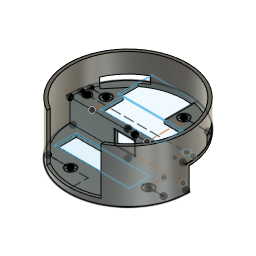
Echo_dev_dock_v1 (Autodesk Fusion 360 design; units mm, degrees)
Autodesk Fusion 360 part; units mm, degrees
sketch "Sketch1" plane through (0, 0, 0) normal (0, 0, 1) x (1, 0, 0)
  circle A0 centre (0, 0) radius 37.65
  line L0 (37.65, 1) -> (-37.65, 1)
  line L1 (-37.65, 1) -> (-37.65, -1)
  line L2 (-37.65, -1) -> (37.65, -1)
  line L3 (37.65, -1) -> (37.65, 1)
  line L4 (37.65, 1) -> (-37.65, -1) construction
  line L5 (-37.65, 1) -> (37.65, -1) construction
  dimension "d1" = 75.3
  dimension "d13" = 75.3
  dimension "d14" = 2
  constraint coincident A0.centre origin
  constraint horizontal L0
  constraint perpendicular L0 L1
  constraint parallel L0 L2
  constraint parallel L1 L3
  constraint coincident L4 A0.centre
  constraint coincident L5 A0.centre
  measures "d1" diameter of A0
  measures "d13" distance of L1.end L2.end
  measures "d14" distance of L0.end L1.end
extrude "Extrude1" add sketch "Sketch1" along normal blind 17 contours A0 L0 L2 | A0 L0 | A0 L2 makes body 1
sketch "Sketch2" plane through (0, 0, 17) normal (0, 0, 1) x (-1, 0, 0)
  circle A0 centre (0, 0) radius 37.65
  line L0 (-37.65, 1) -> (37.65, 1)
  line L1 (37.65, 1) -> (37.65, -1)
  line L2 (37.65, -1) -> (-37.65, -1)
  line L3 (-37.65, -1) -> (-37.65, 1)
  line L4 (-37.65, 1) -> (37.65, -1) construction
  line L5 (37.65, 1) -> (-37.65, -1) construction
  dimension "d4" = 75.3
  dimension "d5" = 2
  constraint horizontal L0
  constraint perpendicular L0 L1
  constraint parallel L0 L2
  constraint parallel L1 L3
  constraint coincident L4 A0.centre
  constraint coincident L5 A0.centre
  constraint coincident A0.centre origin
  measures "d4" distance of L1.end L2.end
  measures "d5" distance of L0.end L1.end
ref_plane "WorkPlane3" through (0, 19.325, 0) normal (0, 0, 1) x (-1, 0, 0)
extrude "Extrude2" cut sketch "Sketch2" against normal blind 15 contours A0 L0 bodies 1
ref_plane "WorkPlane1" through (0, 19.325, 0) normal (0, 0, 1) x (-1, 0, 0)
sketch "Sketch3" plane through (0, 19.325, 0) normal (0, 0, 1) x (1, 0, 0)
ref_plane "WorkPlane2" through (0, 19.325, 0) normal (0, 0, 1) x (-1, 0, 0)
sketch "Sketch4" plane through (0, 19.325, 0) normal (0, 0, 1) x (1, 0, 0)
sketch "Sketch5" plane through (0, 19.325, 0) normal (0, 0, 1) x (1, 0, 0)
ref_plane "WorkPlane4" through (0, 19.325, 0) normal (0, 0, 1) x (-1, 0, 0)
sketch "Sketch6" plane through (0, 19.325, 0) normal (0, 0, 1) x (1, 0, 0)
  line L0 (37.65, -18.3) -> (-37.65, -18.3)
  line L1 (-37.65, -18.3) -> (-37.65, -20.3)
  line L2 (-37.65, -20.3) -> (37.65, -20.3)
  line L3 (37.65, -20.3) -> (37.65, -18.3)
  line L4 (37.65, -18.3) -> (-37.65, -20.3) construction
  line L5 (-37.65, -18.3) -> (37.65, -20.3) construction
  point P0 (0, -19.3)
  dimension "d12" = 75.3
  constraint horizontal L0
  constraint perpendicular L0 L1
  constraint parallel L0 L2
  constraint parallel L1 L3
  constraint coincident L4 P0
  constraint coincident L5 P0
  measures "d12" distance of L1.end L2.end
extrude "Extrude3" cut sketch "Sketch1" along normal blind 15 contours A0 L0 bodies 1
sketch "Sketch8" plane through (0, 0, 2) normal (0, 0, 1) x (-1, 0, 0)
  arc A0 (37.6367, 1) -> (-37.6367, 1) centre (0, 0) ccw
  line L0 (-37.6367, 1) -> (37.6367, 1)
  line L1 (0, 37.65) -> (0, 26.65) construction
  line L2 (0, 26.65) -> (26.5951, 26.65) construction
  line L3 (26.5951, 26.65) -> (11.5951, 26.65) construction
  circle A1 centre (11.5951, 26.65) radius 3.25
  line L4 (-24.8259, 1) -> (-24.8259, 12) construction
  line L5 (-24.8259, 12) -> (-35.6864, 12) construction
  line L6 (-35.6864, 12) -> (-25.6864, 12) construction
  circle A2 centre (-25.6864, 12) radius 3.25
  line L7 (29.3465, 5.0561) -> (-19.5755, 5.0561)
  line L8 (-19.5755, 5.0561) -> (-19.5755, 18.7987)
  line L9 (-19.5755, 18.7987) -> (29.3465, 18.7987)
  line L10 (29.3465, 18.7987) -> (29.3465, 5.0561)
  dimension "d22" = 11
  dimension "d23" = 15
  dimension "d24" = 6.5
  dimension "d27" = 11
  dimension "d28" = 10
  dimension "d29" = 6.5
  constraint midpoint A0 L1.start
  constraint vertical L1
  constraint coincident A0 L2.end
  constraint perpendicular L1 L2
  constraint perpendicular L1 L3
  constraint coincident L3.end A1.centre
  constraint coincident L0 L4.start
  constraint perpendicular L0 L4
  constraint coincident A0 L5.end
  constraint perpendicular L4 L5
  constraint parallel L5 L6
  constraint coincident L6.end A2.centre
  constraint horizontal L7
  constraint vertical L8
  constraint horizontal L9
  constraint vertical L10
  measures "d22" distance of L1.start L1.end
  measures "d23" distance of L2.end L3.end
  measures "d24" diameter of A1
  measures "d27" distance of L4.start L4.end
  measures "d28" distance of L5.end L6.end
  measures "d29" diameter of A2
extrude "Extrude5" cut sketch "Sketch8" against normal blind 2 contours A1 bodies 1
extrude "Extrude6" cut sketch "Sketch8" against normal blind 2 contours A2 bodies 1
sketch "Sketch9" plane through (0, 0, 17) normal (0, 0, 1) x (-1, 0, 0)
  line L0 (37.6367, 1) -> (-37.6367, 1)
  arc A0 (-37.6367, 1) -> (37.6367, 1) centre (0, 0) ccw
  line L1 (22.8923, 1) -> (22.8923, -11) construction
  line L2 (22.8923, -11) -> (36.0073, -11) construction
  line L3 (36.0073, -11) -> (25.5073, -11) construction
  circle A1 centre (25.5073, -11) radius 3.25
  line L4 (-13.6951, 1) -> (-13.6951, -25) construction
  line L5 (-13.6951, -25) -> (-28.1518, -25) construction
  line L6 (-28.1518, -25) -> (-12.1518, -25) construction
  circle A2 centre (-12.1518, -25) radius 3.25
  line L7 (-7.1518, -17) -> (22.9994, -17)
  line L8 (22.9994, -17) -> (22.9994, -39)
  line L9 (22.9994, -39) -> (-7.1518, -39)
  line L10 (-7.1518, -39) -> (-7.1518, -17)
  line L11 (-32.0746, 1) -> (-32.0746, -6) construction
  line L12 (-32.0746, -6) -> (37.1688, -6) construction
  line L13 (-37.1688, -6) -> (-33.1688, -6) construction
  line L14 (37.1688, -6) -> (33.1688, -6) construction
  circle A3 centre (33.1688, -6) radius 2.5
  circle A4 centre (-33.1688, -6) radius 2.5
  line L15 (20.1342, -17) -> (-19.2393, -17)
  line L16 (-19.2393, -17) -> (-19.2393, -2)
  line L17 (-19.2393, -2) -> (20.1342, -2)
  line L18 (20.1342, -2) -> (20.1342, -17)
  arc A5 (-39.636, 1.0531) -> (39.636, 1.0531) centre (0, 0) ccw
  line L19 (-39.636, 1.0531) -> (-37.6367, 1)
  line L20 (39.636, 1.0531) -> (37.6367, 1)
  dimension "d32" = 12
  dimension "d33" = 10.5
  dimension "d34" = 6.5
  dimension "d37" = 26
  dimension "d38" = 16
  dimension "d39" = 6.5
  dimension "d46" = 5
  dimension "d53" = 7
  dimension "d54" = 4
  dimension "d55" = 4
  dimension "d56" = 5
  dimension "d57" = 5
  dimension "d66" = 2
  constraint coincident L0 L1.start
  constraint perpendicular L0 L1
  constraint coincident A0 L2.end
  constraint perpendicular L1 L2
  constraint parallel L2 L3
  constraint coincident L3.end A1.centre
  constraint coincident L0 L4.start
  constraint perpendicular L0 L4
  constraint coincident A0 L5.end
  constraint perpendicular L4 L5
  constraint parallel L5 L6
  constraint coincident L6.end A2.centre
  constraint horizontal L7
  constraint vertical L8
  constraint horizontal L9
  constraint vertical L10
  constraint coincident L0 L11.start
  constraint perpendicular L0 L11
  constraint coincident A0 L12.end
  constraint perpendicular L1 L12
  constraint coincident A0 L13.start
  constraint perpendicular L11 L13
  constraint parallel L12 L14
  constraint coincident L14.end A3.centre
  constraint coincident L13.end A4.centre
  constraint horizontal L15
  constraint vertical L16
  constraint horizontal L17
  constraint vertical L18
  constraint coincident L7 L15.start
  constraint coincident L0.end A0.start
  constraint coincident L0.start A0.end
  measures "d32" distance of L1.start L1.end
  measures "d33" distance of L2.end L3.end
  measures "d34" diameter of A1
  measures "d37" distance of L4.start L4.end
  measures "d38" distance of L5.end L6.end
  measures "d39" diameter of A2
  measures "d46" distance of L6.end L10
  measures "d53" distance of L11.start L11.end
  measures "d54" distance of L13.start L13.end
  measures "d55" distance of L12.end L14.end
  measures "d56" diameter of A3
  measures "d57" diameter of A4
extrude "Extrude8" cut sketch "Sketch9" against normal blind 2 contours A2 bodies 1
extrude "Extrude7" cut sketch "Sketch9" against normal blind 2 contours A1 bodies 1
extrude "Extrude11" cut sketch "Sketch9" against normal blind 2 contours A0 L7 L8 L10 L15 | L7 L15 L16 L17 L18 bodies 1
extrude "Extrude12" cut sketch "Sketch8" against normal blind 2 contours L7 L8 L9 L10 bodies 1
extrude "Extrude14" cut sketch "Sketch9" against normal blind 2 contours A3 | A4 bodies 1
extrude "Extrude10" cut sketch "Sketch8" against normal blind 2 contours L7 L8 L9 L10 bodies 1
sketch "Sketch10" plane through (0, -1, 0) normal (0, -1, 0) x (1, 0, 0)
  line L0 (37.6367, 17) -> (-37.6367, 17)
  line L1 (-37.6367, 17) -> (-37.6367, 2)
  line L2 (-37.6367, 2) -> (37.6367, 2)
  line L3 (37.6367, 2) -> (37.6367, 17)
  line L4 (37.6367, 5.0179) -> (5.6367, 5.0179) construction
  line L5 (5.6367, 5.0179) -> (5.6367, 17) construction
  line L6 (5.6367, 17) -> (5.6367, 13.5) construction
  line L7 (5.6367, 13.5) -> (-7.8633, 13.5)
  line L8 (-7.8633, 13.5) -> (-7.8633, 4.5)
  line L9 (-7.8633, 4.5) -> (5.6367, 4.5)
  line L10 (5.6367, 4.5) -> (5.6367, 13.5)
  dimension "d60" = 32
  dimension "d61" = 3.5
  dimension "d62" = 13.5
  dimension "d63" = 9
  constraint coincident L3 L4.start
  constraint perpendicular L3 L4
  constraint coincident L0 L5.end
  constraint perpendicular L0 L5
  constraint perpendicular L0 L6
  constraint horizontal L7
  constraint vertical L8
  constraint horizontal L9
  constraint vertical L10
  measures "d60" distance of L4.start L4.end
  measures "d61" distance of L5.end L6.end
  measures "d62" distance of L6.end L7.end
  measures "d63" distance of L6.end L9.end
extrude "Extrude15" cut sketch "Sketch10" against normal blind 2 contours L7 L8 L9 L10 bodies 1
extrude "Extrude16" add sketch "Sketch9" along normal blind 15 separate body contours A0 L10 A5 L19 makes body 2
extrude "Extrude17" add sketch "Sketch9" against normal blind 2 contours A0 L10 A5 L19 bodies 1 2
extrude "Extrude18" add sketch "Sketch9" along normal blind 15 separate body contours A0 L8 A5 L20 | A0 L8 L9 L10 A5 | L9 A5 makes body 3
extrude "Extrude19" add sketch "Sketch9" against normal blind 2 contours A0 L8 A5 L20 | A0 L8 L9 L10 A5 | L9 A5 bodies 1 3
sketch "Sketch11" plane through (0, 0, 0) normal (0, 0, -1) x (1, 0, 0)
  line L0 (19.5755, 18.7987) -> (19.5755, 5.0561)
  line L1 (19.5755, 5.0561) -> (-29.3465, 5.0561)
  line L2 (-29.3465, 5.0561) -> (-29.3465, 18.7987)
  line L3 (-29.3465, 18.7987) -> (19.5755, 18.7987)
  circle A0 centre (25.6864, 12) radius 3.25
  circle A1 centre (-11.5951, 26.65) radius 3.25
  line L4 (-37.6367, -1) -> (37.6367, -1)
  arc A2 (37.6367, -1) -> (-37.6367, -1) centre (0, 0) ccw
  arc A3 (39.636, -1.0531) -> (-39.636, -1.0531) centre (0, 0) ccw
  line L5 (39.636, -1.0531) -> (37.6367, -1)
  line L6 (-39.636, -1.0531) -> (-37.6367, -1)
  dimension "d75" = 2
  constraint coincident L4.end A2.start
  constraint coincident L4.start A2.end
extrude "Extrude20" add sketch "Sketch11" against normal blind 32 contours A2 A3 L5 L6 bodies 1
extrude "Extrude21" cut sketch "Sketch10" along normal blind 39 contours L7 L8 L9 L10 bodies 1
ref_plane "WorkPlane5" through (0, -40, 9.5) normal (0, -1, 0) x (1, 0, 0)
sketch "Sketch12" plane through (0, -40, 9.5) normal (0, -1, 0) x (1, 0, 0)
  line L0 (-19.6239, 23.7684) -> (17.5591, 23.7684)
  line L1 (17.5591, 23.7684) -> (17.5591, -6)
  line L2 (17.5591, -6) -> (-19.6239, -6)
  line L3 (-19.6239, -6) -> (-19.6239, 23.7684)
  constraint horizontal L0
  constraint vertical L1
  constraint horizontal L2
  constraint vertical L3
extrude "Extrude22" cut sketch "Sketch12" against normal blind 9 bodies 1
ref_plane "WorkPlane6" through (32.4794, 22.7423, 23.0666) normal (0.819152, 0.573576, 0) x (0.573576, -0.819152, 0)
sketch "Sketch13" plane through (32.4794, 22.7423, 23.0666) normal (0.819152, 0.573576, 0) x (0.573576, -0.819152, 0)
  line L0 (7, 6) -> (-3, 6)
  line L1 (-3, 6) -> (-3, 0)
  line L2 (-3, 0) -> (7, 0)
  line L3 (7, 0) -> (7, 6)
  dimension "d84" = 10
  dimension "d89" = 6
  constraint horizontal L0
  constraint vertical L1
  constraint horizontal L2
  constraint vertical L3
  measures "d84" distance of L0.start L0.end
  measures "d89" distance of L0.end L1.end
extrude "Extrude23" cut sketch "Sketch13" against normal blind 3 bodies 1
extrude "Extrude24" add 6 faces at (-22.6844, -30.7905, 32) (20.5223, -32.2828, 32) (8.8959, 37.8769, 32) (-38.9777, -0.5792, 32) (38.9737, 0.8014, 32) (-29.4892, 24.3577, 32) along direction (0, 0, 1) blind 3 on bodies 1 bodies 1
ref_plane "WorkPlane7" through (-30.3737, 25.4865, 24.2625) normal (-0.766044, 0.642788, 0) x (0.642788, 0.766044, 0)
sketch "Sketch14" plane through (-30.3737, 25.4865, 24.2625) normal (-0.766044, 0.642788, 0) x (0.642788, 0.766044, 0)
  line L0 (-10.26, 7.2753) -> (13.74, 7.2753)
  line L1 (13.74, 7.2753) -> (13.74, 2.2753)
  line L2 (13.74, 2.2753) -> (-10.26, 2.2753)
  line L3 (-10.26, 2.2753) -> (-10.26, 7.2753)
  dimension "d91" = 24
  dimension "d92" = 5
  constraint horizontal L0
  constraint vertical L1
  constraint horizontal L2
  constraint vertical L3
  measures "d91" distance of L1.end L2.end
  measures "d92" distance of L0.start L2.end
extrude "Extrude25" cut sketch "Sketch14" against normal blind 6 bodies 1
